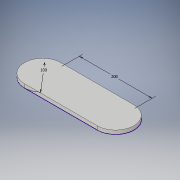
# Autodesk Inventor part: test
Saved by Autodesk Inventor 2019 (Build 230136000, 136)
## iProperties
Created: 2021-02-06
Part Number: test
Material: 一般
Document SubType Name: Modeling
Designer: wasd5
Density: 1 g/cm^3
Appearance: 預設
Author: wasd5
Autodesk Inventor part; units mm, degrees
ref_plane "YZ Plane" through (0, 0, 0) normal (1, 0, 0) x (0, 1, 0)
ref_plane "XZ Plane" through (0, 0, 0) normal (0, 1, 0) x (-1, 0, 0)
ref_plane "XY Plane" through (0, 0, 0) normal (0, 0, 1) x (1, 0, 0)
sketch "草圖1" plane through (0, 0, 0) normal (0, 1, 0) x (-1, 0, 0)
  arc A0 (0, -50) -> (0, 50) centre (0, 0) ccw
  line L0 (0, -50) -> (-200, -50)
  line L1 (-200, -50) -> (-200, 50) construction
  line L2 (-200, 50) -> (0, 50)
  line L3 (0, 50) -> (0, -50) construction
  arc A1 (-200, 50) -> (-200, -50) centre (-200, 0) ccw
  dimension "diameter" = 100
  dimension "center_length" = 200
  constraints: 8 end point, 4 point on circle, 2 centre point, 2 parallel, 2 tangent, 1 coincident, 1 horizontal, 1 midpoint, 1 perpendicular
  measures "diameter" diameter of A0
  measures "center_length" distance of L0.start L0.end
extrude "thickness" add sketch "草圖1" along normal blind 10
